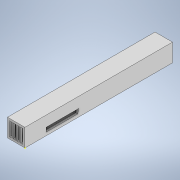
# Autodesk Inventor part: box
Saved by Autodesk Inventor 2021 (Build 250183000, 183)
## iProperties
Created: 2021-06-29
Part Number: box
Material: Generic
Document SubType Name: Modeling
Designer: newic
Density: 1 g/cm^3
Appearance: Default
Author: newic
Autodesk Inventor part; units mm, degrees
ref_plane "YZ Plane" through (0, 0, 0) normal (1, 0, 0) x (0, 1, 0)
ref_plane "XZ Plane" through (0, 0, 0) normal (0, 1, 0) x (-1, 0, 0)
ref_plane "XY Plane" through (0, 0, 0) normal (0, 0, 1) x (1, 0, 0)
sketch "Sketch1" plane through (0, 0, 0) normal (0, 1, 0) x (-1, 0, 0)
  line L0 (0, 0) -> (105.41, 0)
  line L1 (105.41, 0) -> (105.41, 863.6)
  line L2 (105.41, 863.6) -> (0, 863.6)
  line L3 (0, 863.6) -> (0, 0)
  dimension "d0" = 105.41
  dimension "d1" = 863.6
  constraints: 8 end point, 2 parallel, 1 horizontal, 1 perpendicular
  measures "d0" distance of L2.end L1.end
  measures "d1" distance of L1.end L0.end
extrude "Extrusion1" add sketch "Sketch1" along normal blind 12.7
sketch "Sketch2" plane through (0, 12.7, 0) normal (0, 1, 0) x (1, 0, 0)
  line L0 (0, 0) -> (-105.41, 0) projected
  line L1 (0, 0) -> (-12.7, 0)
  line L2 (-12.7, 0) -> (-12.7, 12.7)
  line L3 (-12.7, 12.7) -> (0, 12.7)
  line L4 (0, 12.7) -> (0, 0)
  line L5 (-105.41, 0) -> (-105.41, -863.6) projected
  line L6 (0, 12.7) -> (-105.41, 12.7)
  line L7 (-105.41, 12.7) -> (-105.41, 0)
  line L8 (-105.41, 0) -> (0, 0)
  line L9 (0, 0) -> (0, 12.7)
  line L10 (0, -863.6) -> (0, 0) projected
  line L11 (0, -863.6) -> (-105.41, -863.6)
  line L12 (-105.41, -863.6) -> (-105.41, -876.3)
  line L13 (-105.41, -876.3) -> (0, -876.3)
  line L14 (0, -876.3) -> (0, -863.6)
  line L15 (-105.41, -863.6) -> (-92.71, -863.6)
  line L16 (-92.71, -863.6) -> (-92.71, 12.7)
  line L17 (-92.71, 12.7) -> (-105.41, 12.7)
  line L18 (-105.41, 12.7) -> (-105.41, -863.6)
  line L19 (0, 12.7) -> (-12.7, 12.7)
  line L20 (-12.7, 12.7) -> (-12.7, -876.3)
  line L21 (-12.7, -876.3) -> (0, -876.3)
  line L22 (0, -876.3) -> (0, 12.7)
  point P0 (-12.7, -863.6)
  point P1 (-92.71, 0)
  dimension "d4" = 12.7
  dimension "d5" = 12.7
  dimension "d6" = 12.7
  dimension "d7" = 12.7
  dimension "d8" = 12.7
  constraints: 40 end point, 10 parallel, 5 horizontal, 5 perpendicular, 3 point on line
  measures "d4" distance of L2.end L3.end
  measures "d5" distance of L1.end L2.end
  measures "d6" distance of L12.end L11.end
  measures "d7" distance of L17.end L16.end
  measures "d8" distance of L21.end L20.end
extrude "Extrusion2" add sketch "Sketch2" along normal blind 95.25 and the other way blind 12.7 contours L10 L11 L20 L0 | L0 L2 L3 L4 | L0 L16 L6 L2 | L14 L13 L20 L11 | L16 L11 L5 L0 | L0 L7 L6 L16 | L20 L13 L12 L11
sketch "Sketch3" plane through (-105.41, 107.95, 876.3) normal (0, 0, 1) x (1, 0, 0)
  line L0 (12.7, -95.25) -> (92.71, -95.25) projected
  line L1 (12.7, -95.25) -> (12.7, 0) projected
  line L2 (92.71, -95.25) -> (92.71, 0) projected
  line L3 (92.71, -95.25) -> (77.47, -95.25)
  line L4 (77.47, -95.25) -> (77.47, -12.7)
  line L5 (77.47, -12.7) -> (92.71, -12.7)
  line L6 (92.71, -12.7) -> (92.71, -95.25)
  line L7 (12.7, -95.25) -> (27.94, -95.25)
  line L8 (27.94, -95.25) -> (27.94, -12.7)
  line L9 (27.94, -12.7) -> (12.7, -12.7)
  line L10 (12.7, -12.7) -> (12.7, -95.25)
  line L11 (27.94, -95.25) -> (34.29, -95.25)
  line L12 (34.29, -95.25) -> (34.29, -12.7)
  line L13 (34.29, -12.7) -> (27.94, -12.7)
  line L14 (27.94, -12.7) -> (27.94, -95.25)
  line L15 (77.47, -95.25) -> (71.12, -95.25)
  line L16 (71.12, -95.25) -> (71.12, -12.7)
  line L17 (71.12, -12.7) -> (77.47, -12.7)
  line L18 (77.47, -12.7) -> (77.47, -95.25)
  line L19 (34.29, -95.25) -> (49.53, -95.25)
  line L20 (49.53, -95.25) -> (49.53, -12.7)
  line L21 (49.53, -12.7) -> (34.29, -12.7)
  line L22 (34.29, -12.7) -> (34.29, -95.25)
  line L23 (71.12, -95.25) -> (55.88, -95.25)
  line L24 (55.88, -95.25) -> (55.88, -12.7)
  line L25 (55.88, -12.7) -> (71.12, -12.7)
  line L26 (71.12, -12.7) -> (71.12, -95.25)
  point P0 (105.41, -107.95)
  dimension "d13" = 15.24
  dimension "d14" = 82.55
  dimension "d15" = 15.24
  dimension "d16" = 6.35
  dimension "d17" = 6.35
  dimension "d18" = 15.24
  dimension "d19" = 15.24
  constraints: 48 end point, 12 parallel, 6 horizontal, 6 perpendicular, 4 point on line
  measures "d13" distance of L4.end L5.end
  measures "d14" distance of L3.end L4.end
  measures "d15" distance of L9.end L8.end
  measures "d16" distance of L13.end L12.end
  measures "d17" distance of L16.end L17.end
  measures "d18" distance of L21.end L20.end
  measures "d19" distance of L24.end L25.end
extrude "Extrusion3" cut sketch "Sketch3" against normal blind 95.25 contours L1 L9 L8 L0 | L24 L25 L16 L0 | L12 L21 L20 L0 | L4 L5 L2 L0
sketch "Sketch5" plane through (-105.41, 107.95, 876.3) normal (0, 0, 1) x (1, 0, 0)
  line L0 (71.12, -95.25) -> (55.88, -95.25) projected
  line L1 (55.88, -95.25) -> (55.88, -12.7) projected
  line L2 (55.88, -12.7) -> (71.12, -12.7) projected
  line L3 (71.12, -12.7) -> (71.12, -95.25) projected
  line L4 (49.53, -95.25) -> (34.29, -95.25) projected
  line L5 (34.29, -95.25) -> (34.29, -12.7) projected
  line L6 (34.29, -12.7) -> (49.53, -12.7) projected
  line L7 (49.53, -12.7) -> (49.53, -95.25) projected
  line L8 (92.71, -95.25) -> (77.47, -95.25) projected
  line L9 (77.47, -95.25) -> (77.47, -12.7) projected
  line L10 (77.47, -12.7) -> (92.71, -12.7) projected
  line L11 (92.71, -12.7) -> (92.71, -95.25) projected
  line L12 (27.94, -95.25) -> (12.7, -95.25) projected
  line L13 (12.7, -95.25) -> (12.7, -12.7) projected
  line L14 (12.7, -12.7) -> (27.94, -12.7) projected
  line L15 (27.94, -12.7) -> (27.94, -95.25) projected
  line L16 (105.41, -107.95) -> (105.41, 0) projected
  line L17 (0, 0) -> (105.41, 0) projected
  line L18 (0, -107.95) -> (0, 0) projected
  line L19 (105.41, -107.95) -> (0, -107.95) projected
  line L20 (92.71, 0) -> (12.7, 0) projected
  circle A0 centre (52.705, 26.3525) radius 26.3525
  dimension "d40" = 52.705
  constraints: 1 centre point
  measures "d40" diameter of A0
extrude "Extrusion4" add sketch "Sketch5" against normal blind 1270 contours A0
sketch "Sketch6" plane through (0, 0, -12.7) normal (1, 0, 0) x (0, 0, -1)
  line L0 (0, 0) -> (-889, 0) projected
  line L1 (-444.5, 0) -> (-444.5, 160.655)
  line L2 (-889, 160.655) -> (381, 160.655) projected
  line L3 (-444.5, 160.655) -> (-444.5, 167.005)
  line L4 (-444.5, 0) -> (-444.5, -6.35)
  line L5 (-444.5, 167.005) -> (-428.625, 167.005)
  line L6 (-428.625, 167.005) -> (-460.375, 167.005)
  line L7 (-428.625, 167.005) -> (-460.375, 167.005)
  line L8 (-460.375, 167.005) -> (-460.375, -6.35)
  line L9 (-460.375, -6.35) -> (-428.625, -6.35)
  line L10 (-428.625, -6.35) -> (-428.625, 167.005)
  line L11 (-889, 0) -> (-793.75, 0)
  line L12 (0, 107.95) -> (0, 0) projected
  line L13 (0, 0) -> (-95.25, 0)
  line L14 (-95.25, 0) -> (-95.25, -6.35)
  line L15 (-793.75, 0) -> (-793.75, -6.35)
  line L16 (-793.75, -6.35) -> (-762, -6.35)
  line L17 (-762, -6.35) -> (-762, 167.005)
  line L18 (-762, 167.005) -> (-793.75, 167.005)
  line L19 (-793.75, 167.005) -> (-793.75, -6.35)
  line L20 (-95.25, -6.35) -> (-127, -6.35)
  line L21 (-127, -6.35) -> (-127, 167.005)
  line L22 (-127, 167.005) -> (-95.25, 167.005)
  line L23 (-95.25, 167.005) -> (-95.25, -6.35)
  line L24 (-111.125, 167.005) -> (-111.125, -6.35)
  line L25 (-777.875, -6.35) -> (-777.875, 167.005)
  line L26 (-777.875, 79.2503) -> (-762, 79.2503)
  line L27 (-111.125, 68.9503) -> (-95.25, 68.9503)
  line L28 (-451.8389, 167.005) -> (-451.8389, 163.0426)
  circle A0 centre (-444.5, 148.7424) radius 10.8761
  circle A1 centre (-444.5, 11.9126) radius 11.9126
  line L29 (-456.4123, 12.0028) -> (-455.3758, 148.8248)
  line L30 (-433.6242, 148.8248) -> (-432.5877, 12.0028)
  line L31 (-127, 12.7) -> (-139.7, 12.7)
  line L32 (-139.7, 12.7) -> (-165.1, 12.7)
  line L33 (-460.375, 21.426) -> (-473.075, 21.426)
  line L34 (0, 107.95) -> (-889, 107.95) projected
  line L35 (-524.7767, 107.95) -> (-524.7767, 0)
  line L36 (-524.7767, 53.975) -> (-485.775, 53.975)
  circle A2 centre (-485.775, 53.975) radius 12.7
  line L37 (-498.475, 0) -> (-498.475, -3.175)
  line L38 (-498.475, -3.175) -> (-473.075, -3.175)
  line L39 (-473.075, -3.175) -> (-473.075, 53.975)
  line L40 (-498.475, 53.975) -> (-498.475, 0)
  line L41 (-694.0635, 0) -> (-694.0635, 19.05)
  line L42 (-762, 19.05) -> (-571.5, 19.05)
  line L43 (-687.1312, 19.05) -> (-687.1312, 44.45)
  line L44 (-762, 44.45) -> (-565.15, 44.45)
  line L45 (-571.5, 19.05) -> (-565.15, 44.45)
  point P0 (-12.7, 0)
  dimension "d25" = 6.35
  dimension "d26" = 6.35
  dimension "d27" = 15.875
  dimension "d28" = 31.75
  dimension "d29" = 95.25
  dimension "d30" = 95.25
  dimension "d31" = 6.35
  dimension "d32" = 6.35
  dimension "d33" = 31.75
  dimension "d34" = 31.75
  dimension "d35" = 3.9624
  dimension "d39" = 23.8252
  dimension "d41" = 12.7
  dimension "d42" = 25.4
  dimension "d43" = 12.7
  dimension "d45" = 19.05
  dimension "d46" = 190.5
  dimension "d47" = 25.4
  dimension "d48" = 196.85
  constraints: 84 end point, 18 point on line, 9 vertical, 8 horizontal, 8 perpendicular, 6 parallel, 6 point on circle, 5 midpoint, 4 tangent, 3 centre point, 1 coincident, 8 other
  measures "d25" distance of L1.end L3.end
  measures "d26" distance of L1.start L4.end
  measures "d27" distance of L3.end L5.end
  measures "d28" distance of L5.end L6.end
  measures "d29" distance of L11.start L11.end
  measures "d30" distance of L12.end L13.end
  measures "d31" distance of L13.end L14.end
  measures "d32" distance of L11.end L15.end
  measures "d33" distance of L18.end L17.end
  measures "d34" distance of L21.end L22.end
  measures "d35" distance of L28.start L28.end
  measures "d39" diameter of A1
  measures "d41" distance of L31.start L31.end
  measures "d42" distance of L31.end L32.end
  measures "d43" distance of L33.start L33.end
  measures "d45" distance of L41.start L41.end
  measures "d46" distance of L42.start L42.end
  measures "d47" distance of L43.start L43.end
  measures "d48" distance of L44.start L44.end
sketch "Sketch7" plane through (-105.41, 0, 876.3) normal (0, 0, 1) x (1, 0, 0)
  point P0 (105.41, 0)
extrude "Extrusion5" cut sketch "Sketch6" against normal blind 15.24 contours L42 L17 L44 L43 | L43 L44 L45 L42
sketch "Sketch8" plane through (0, 107.95, 0) normal (0, 1, 0) x (1, 0, 0)
  line L0 (0, -876.3) -> (0, 12.7) projected
  line L1 (-105.41, 12.7) -> (-105.41, -876.3) projected
  line L2 (0, 12.7) -> (-105.41, 12.7)
  line L3 (-105.41, 12.7) -> (-105.41, -876.3)
  line L4 (-105.41, -876.3) -> (0, -876.3)
  line L5 (0, -876.3) -> (0, 12.7)
  point P0 (0, 0)
  constraints: 8 end point, 2 parallel, 1 horizontal, 1 perpendicular
extrude "Extrusion6" add sketch "Sketch8" against normal blind 12.7
sketch "Sketch9" plane through (-52.705, 134.3025, 876.3) normal (0, 0, 1) x (1, 0, 0)
  line L0 (-52.705, -26.3525) -> (0, -26.3525) projected
  line L1 (-39.5109, -26.3525) -> (301.585, -26.3525)
  line L2 (301.585, -26.3525) -> (301.585, 239.994)
  line L3 (301.585, 239.994) -> (-39.5109, 239.994)
  line L4 (-39.5109, 239.994) -> (-39.5109, -26.3525)
  point P0 (52.705, -134.3025)
  constraints: 8 end point, 2 parallel, 1 horizontal, 1 perpendicular, 1 point on line
extrude "Extrusion7" cut sketch "Sketch9" against normal through all
sketch "Sketch10" plane through (-105.41, 0, 876.3) normal (0, 0, 1) x (1, 0, 0)
  point P0 (105.41, 0)
body "Solid1"
